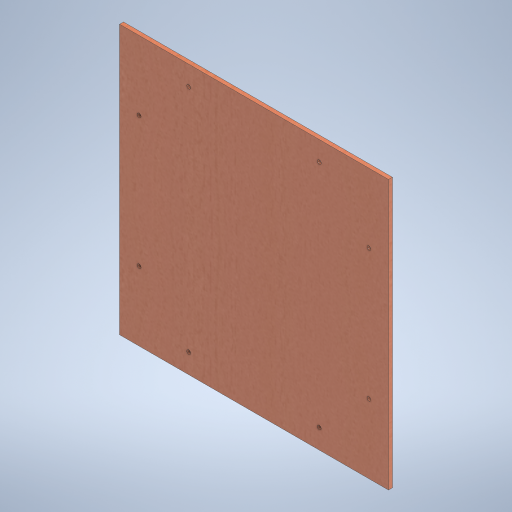
# Autodesk Inventor part: Tapa_Inferior
Saved by Autodesk Inventor 2024 (Build 280153000, 153)
## iProperties
Created: 2024-07-16
Part Number: Tapa_Inferior
Material: Genérico
Document SubType Name: Modeling
Designer: sergi
Density: 1 g/cm^3
Appearance: Valor por defecto
Author: sergi
Autodesk Inventor part; units mm, degrees
ref_plane "YZ Plane" through (0, 0, 0) normal (1, 0, 0) x (0, 1, 0)
ref_plane "XZ Plane" through (0, 0, 0) normal (0, 1, 0) x (-1, 0, 0)
ref_plane "XY Plane" through (0, 0, 0) normal (0, 0, 1) x (1, 0, 0)
sketch "Boceto1" plane through (0, 0, 0) normal (0, 0, 1) x (1, 0, 0)
  line L0 (-103, -100) -> (-103, 103) projected
  line L1 (-100, 103) -> (-100, -100) projected
  line L2 (-103, 103) -> (-100, 103) projected
  line L3 (-100, 103) -> (103, 103) projected
  line L4 (103, 103) -> (103, 100) projected
  line L5 (103, 103) -> (-103, 103)
  line L6 (-103, 103) -> (-103, -100)
  line L7 (-103, -100) -> (103, -100)
  line L8 (103, -100) -> (103, 103)
  line L9 (103, -103) -> (-103, -103)
  line L10 (-103, -103) -> (-103, 103)
  line L11 (-103, 103) -> (103, 103)
  line L12 (103, 103) -> (103, -103)
  line L13 (-103, -100) -> (-100, -100) projected
  point P0 (0, 0)
  constraints: 16 end point, 4 parallel, 2 horizontal, 2 perpendicular
extrude "Extrusión1" add sketch "Boceto1" along normal blind 3
sketch "Boceto2" plane through (0, 0, 3) normal (0, 0, 1) x (1, 0, 0)
  line L0 (51.75, -100) -> (48.25, -100) projected
  line L1 (-48.25, -100) -> (-51.75, -100) projected
  line L2 (50, -100) -> (50, -88)
  line L3 (-50, -100) -> (-50, -88)
  circle A0 centre (50, -88) radius 1.5
  circle A1 centre (-50, -88) radius 1.5
  point P0 (0, 0)
  dimension "d2" = 12
  dimension "d3" = 12
  dimension "d5" = 3
  dimension "d6" = 3
  constraints: 4 end point, 2 centre point, 2 coincident, 2 midpoint, 1 vertical
  measures "d2" distance of L2.start L2.end
  measures "d3" distance of L3.start L3.end
  measures "d5" diameter of A0
  measures "d6" diameter of A1
hole "Agujero1" at (50, -88, 3) at (-50, -88, 3) direction (0, 0, -1) diameter 3 depth 7
pattern_circular "Patrón circular1" count 4 over 360 about axis through (0, 0, -10) along (0, 0, 1) of "Agujero1"
